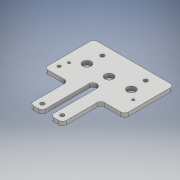
# Autodesk Inventor part: shovel_mount
Saved by Autodesk Inventor 2017.2 (Build 212233000, 233)
## iProperties
Created: 2017-09-14
Part Number: shovel_mount
Material: Generic
Document SubType Name: Modeling
Designer: Nic
Density: 1 g/cm^3
Appearance: Default
Author: Nic
Autodesk Inventor part; units mm, degrees
ref_plane "YZ Plane" through (0, 0, 0) normal (1, 0, 0) x (0, 1, 0)
ref_plane "XZ Plane" through (0, 0, 0) normal (0, 1, 0) x (-1, 0, 0)
ref_plane "XY Plane" through (0, 0, 0) normal (0, 0, 1) x (1, 0, 0)
sketch "Sketch2" plane through (0, 0, 0) normal (0, 0, 1) x (1, 0, 0)
  line L0 (-10.25, -25) -> (-6.25, -25)
  line L1 (-3.25, -22) -> (-3.25, 13)
  line L2 (-0.25, 16) -> (0.25, 16)
  line L3 (3.25, 13) -> (3.25, -22)
  line L4 (6.25, -25) -> (10.25, -25)
  line L5 (29.5, 46) -> (-29.5, 46)
  line L6 (-32.5, 43) -> (-32.5, 9)
  line L7 (0, 0) -> (0, 46) construction
  circle A0 centre (-17.5, 38) radius 1.6
  circle A1 centre (17.5, 38) radius 1.6
  circle A2 centre (-8.05, -20) radius 1.6
  circle A3 centre (8.05, -20) radius 1.6
  line L8 (0, 0) -> (32.5, 0) construction
  arc A4 (-0.25, 16) -> (-3.25, 13) centre (-0.25, 13) ccw
  arc A5 (3.25, 13) -> (0.25, 16) centre (0.25, 13) ccw
  arc A6 (-29.5, 46) -> (-32.5, 43) centre (-29.5, 43) ccw
  arc A7 (32.5, 43) -> (29.5, 46) centre (29.5, 43) ccw
  arc A8 (3.25, -22) -> (6.25, -25) centre (6.25, -22) ccw
  arc A9 (-6.25, -25) -> (-3.25, -22) centre (-6.25, -22) ccw
  circle A10 centre (-27.5, 13) radius 1.3
  line L9 (29.5, 6) -> (16.25, 6)
  line L10 (13.25, 3) -> (13.25, -22)
  line L11 (-29.5, 6) -> (-16.25, 6)
  line L12 (-13.25, 3) -> (-13.25, -22)
  line L13 (32.5, 9) -> (32.5, 43)
  arc A11 (10.25, -25) -> (13.25, -22) centre (10.25, -22) ccw
  arc A12 (-13.25, -22) -> (-10.25, -25) centre (-10.25, -22) ccw
  arc A13 (16.25, 6) -> (13.25, 3) centre (16.25, 3) ccw
  arc A14 (-13.25, 3) -> (-16.25, 6) centre (-16.25, 3) ccw
  arc A15 (29.5, 6) -> (32.5, 9) centre (29.5, 9) ccw
  arc A16 (-32.5, 9) -> (-29.5, 6) centre (-29.5, 9) ccw
  point P0 (-3.25, 16)
  point P1 (3.25, 16)
  point P2 (3.25, -25)
  point P3 (32.5, 6)
  point P4 (13.25, 6)
  point P5 (-13.25, 6)
  point P6 (13.25, -25)
  point P7 (-13.25, -25)
  point P8 (-32.5, 6)
  dimension "d1" = 16.1
  dimension "d3" = 16
  dimension "d4" = 20
  dimension "d5" = 5
  dimension "d6" = 6.5
  dimension "d7" = 3.2
  dimension "d13" = 8
  dimension "d14" = 15
  dimension "d16" = 30
  dimension "d18" = 3.2
  dimension "d19" = 3
  dimension "d20" = 3
  dimension "d23" = 5
  dimension "d24" = 33
  dimension "d25" = 2.6
  dimension "d26" = 32.5
  dimension "d27" = 10
  dimension "d28" = 3
  dimension "d29" = 40
  constraints: 28 end point, 24 point on circle, 24 tangent, 19 point on line, 17 centre point, 10 equal radius, 8 perpendicular, 3 symmetric about line, 2 horizontal, 1 midpoint, 1 vertical, 4 other
  measures "d1" distance of A3.centre A2.centre
  measures "d3" distance between parallel lines of L2 L8
  measures "d4" distance from line of L8 A3.centre
  measures "d5" distance from line of L4 A3.centre
  measures "d6" distance of point (-3.25, 16) point (3.25, 16)
  measures "d7" diameter of A2
  measures "d13" distance from line of L5 A0.centre
  measures "d14" distance from line of L6 A0.centre
  measures "d16" distance between parallel lines of L5 L2
  measures "d18" diameter of A0
  measures "d19" radius of A4
  measures "d20" radius of A6
  measures "d23" distance from line of L6 A10.centre
  measures "d24" distance from line of L5 A10.centre
  measures "d25" diameter of A10
  measures "d26" distance between parallel lines of L13 L7
  measures "d27" distance between parallel lines of L10 L3
  measures "d28" radius of A11
  measures "d29" distance between parallel lines of L5 L9
extrude "Extrusion1" add sketch "Sketch2" along normal blind 3.175
sketch "Sketch3" plane through (0, 0, 0) normal (0, 0, -1) x (-1, 0, 0)
  circle A0 centre (0, 26) radius 3.4
  circle A1 centre (18, 26) radius 3.4
  circle A2 centre (-18, 26) radius 3.4
  line L0 (-29.5, 46) -> (29.5, 46) projected
  line L1 (-32.5, 9) -> (-32.5, 43) construction
  line L2 (-32.5, 26) -> (32.5, 26) construction
  line L3 (32.5, 43) -> (32.5, 9) construction
  line L4 (-18, 26) -> (18, 26) construction
  line L5 (-29.5, 46) -> (29.5, 46) construction
  line L6 (0, 46) -> (0, 26) construction
  circle A3 centre (-26, 19.5) radius 1
  circle A4 centre (26, 19.5) radius 1
  line L7 (0, 26) -> (0, 46) construction
  point P0 (0, 0)
  dimension "d30" = 6.8
  dimension "d34" = 18
  dimension "d35" = 18
  dimension "d38" = 52
  dimension "d39" = 6.5
  dimension "d40" = 2
  constraints: 8 end point, 5 centre point, 4 midpoint, 2 collinear, 2 equal radius, 1 horizontal, 1 perpendicular, 1 other
  measures "d30" diameter of A0
  measures "d34" distance of L4.end L6.end
  measures "d35" distance of L4.start L6.end
  measures "d38" distance of A4.centre A3.centre
  measures "d39" distance from line of L2 A3.centre
  measures "d40" diameter of A3
extrude "Extrusion2" cut sketch "Sketch3" against normal up to next
body "Solid1"
